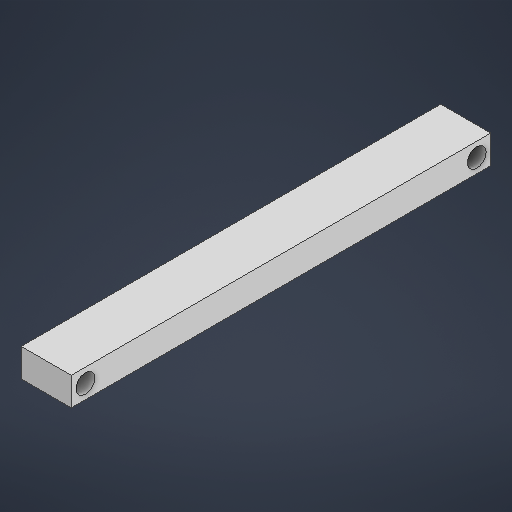
# Autodesk Inventor part: suport4_pcb_temp
Saved by Autodesk Inventor 2026.1 (Build 301233000, 233)
## iProperties
Created: 2025-09-30
Part Number: suport4_pcb_temp
Material: Generic
Document SubType Name: Modeling
Designer: emanuel
Density: 1 g/cm^3
Appearance: Default
Author: emanuel
Autodesk Inventor part; units mm, degrees
ref_plane "YZ Plane" through (0, 0, 0) normal (1, 0, 0) x (0, 1, 0)
ref_plane "XZ Plane" through (0, 0, 0) normal (0, 1, 0) x (-1, 0, 0)
ref_plane "XY Plane" through (0, 0, 0) normal (0, 0, 1) x (1, 0, 0)
sketch "Sketch1" plane through (0, 0, 0) normal (0, 1, 0) x (-1, 0, 0)
  line L0 (0, 0) -> (8, 0)
  line L1 (8, 0) -> (8, -67)
  line L2 (8, -67) -> (0, -67)
  line L3 (0, -67) -> (0, 0)
  dimension "d0" = 8
  dimension "d1" = 67
  constraints: 8 end point, 2 parallel, 1 horizontal, 1 perpendicular
  measures "d0" distance of L1.end L2.end
  measures "d1" distance of L0.end L1.end
extrude "Extrusion1" add sketch "Sketch1" along normal blind 4.5
sketch "Sketch2" plane through (0, 0, 0) normal (1, 0, 0) x (0, 0, -1)
  line L0 (0, 0) -> (0, 4.5) projected
  line L1 (0, 4.5) -> (2.25, 4.5)
  line L2 (2.25, 4.5) -> (2.25, 2.25)
  line L3 (2.25, 2.25) -> (0, 2.25)
  line L4 (0, 2.25) -> (0, 4.5)
  circle A0 centre (2.25, 2.25) radius 1.5
  line L5 (67, 0) -> (67, 4.5) projected
  line L6 (67, 4.5) -> (64.75, 4.5)
  line L7 (64.75, 4.5) -> (64.75, 2.25)
  line L8 (64.75, 2.25) -> (67, 2.25)
  line L9 (67, 2.25) -> (67, 4.5)
  circle A1 centre (64.75, 2.25) radius 1.5
  dimension "d4" = 2.25
  dimension "d5" = 2.25
  dimension "d6" = 3
  dimension "d7" = 2.25
  dimension "d8" = 2.25
  dimension "d9" = 3
  constraints: 16 end point, 4 parallel, 2 centre point, 2 coincident, 2 horizontal, 2 perpendicular
  measures "d4" distance of L2.end L3.end
  measures "d5" distance of L1.end L2.end
  measures "d6" diameter of A0
  measures "d7" distance of L8.end L7.end
  measures "d8" distance of L7.end L6.end
  measures "d9" diameter of A1
extrude "Extrusion2" cut sketch "Sketch2" against normal blind 10 contours A0 L2 L3 | L3 L2 A0 | A1 L7 L8 | L8 L7 A1
body "Solid1"
